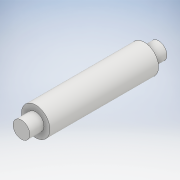
# Autodesk Inventor part: Pok Mk3 Support
Saved by Autodesk Inventor 2018.2 (Build 222227000, 227)
## iProperties
Created: 2018-02-12
Part Number: Pok Mk3 Support
Material: ABS Plastic
Document SubType Name: Modeling
Designer: Moochster
Density: 1.06 g/cm^3
Appearance: Smooth - White
Author: Moochster
Autodesk Inventor part; units mm, degrees
ref_plane "YZ Plane" through (0, 0, 0) normal (1, 0, 0) x (0, 1, 0)
ref_plane "XZ Plane" through (0, 0, 0) normal (0, 1, 0) x (-1, 0, 0)
ref_plane "XY Plane" through (0, 0, 0) normal (0, 0, 1) x (1, 0, 0)
sketch "Sketch1" plane through (0, 0, 0) normal (0, 0, 1) x (1, 0, 0)
  line L0 (0, 0) -> (0, 38.5)
  line L1 (0, 38.5) -> (2.35, 38.5)
  line L2 (2.35, 38.5) -> (2.35, 34.5)
  line L3 (2.35, 34.5) -> (4, 34.5)
  line L4 (4, 34.5) -> (4, 4)
  line L5 (4, 4) -> (2.35, 4)
  line L6 (2.35, 4) -> (2.35, 0)
  line L7 (2.35, 0) -> (0, 0)
  dimension "d0" = 30.5
  dimension "d1" = 8
  dimension "d2" = 4.7
  dimension "d3" = 4
  dimension "d4" = 4
  constraints: 16 end point, 5 perpendicular, 2 point on line, 1 horizontal, 1 vertical
  measures "d0" distance of L3.end L4.end
  measures "d1" diameter of L4 L0
  measures "d2" diameter of L2 L0
  measures "d3" distance of L1.end L2.end
  measures "d4" distance of L5.end L6.end
revolve "Revolution1" add sketch "Sketch1" angle 360 about axis through (0, 0, 0) along (0, 1, 0)
body "Solid1"
